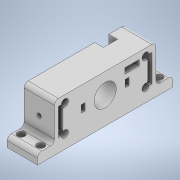
# Autodesk Inventor part: Y_motor_mount
Saved by Autodesk Inventor 2020 (Build 240168000, 168)
## iProperties
Created: 2022-04-26
Part Number: Y_motor_mount
Material: Ogólny
Document SubType Name: Modeling
Designer: mikoma
Density: 1 g/cm^3
Appearance: Domyślna
Mass: 413.903 g
Surface Area: 679.548 cm^2
Volume: 413.903 cm^3
Author: mikoma
Autodesk Inventor part; units mm, degrees
ref_plane "YZ Plane" through (0, 0, 0) normal (1, 0, 0) x (0, 1, 0)
ref_plane "XZ Plane" through (0, 0, 0) normal (0, 1, 0) x (-1, 0, 0)
ref_plane "XY Plane" through (0, 0, 0) normal (0, 0, 1) x (1, 0, 0)
sketch "Szkic1" plane through (0, 0, 0) normal (1, 0, 0) x (0, 1, 0)
  circle A0 centre (0, 0) radius 16.5
  arc A1 (16.0869, 63.5) -> (15.2371, 62.2084) centre (20, 60) ccw construction
  arc A2 (-20.25, 65.244) -> (-15.2371, 62.2084) centre (-20, 60) ccw
  line L0 (20.25, 69.5) -> (-20.25, 69.5)
  line L1 (-20.25, 69.5) -> (-20.25, 65.244)
  line L2 (-20.25, 63.5) -> (-16.0869, 63.5) construction
  line L3 (20.25, 63.5) -> (20.25, 65.244) construction
  line L4 (16.0869, 63.5) -> (20.25, 63.5) construction
  line L5 (20.25, 65.244) -> (20.25, 69.5)
  line L6 (-20.25, 65.244) -> (-20.25, 63.5) construction
  line L7 (-16.0869, 63.5) -> (-13, 63.5) construction
  arc A3 (20.25, 65.244) -> (16.0869, 63.5) centre (20, 60) ccw construction
  arc A4 (-16.0869, 63.5) -> (-20.25, 65.244) centre (-20, 60) ccw construction
  line L8 (-15.2371, 62.2084) -> (-13, 63.5)
  line L9 (13, 63.5) -> (15.2371, 62.2084)
  arc A5 (15.2371, 62.2084) -> (20.25, 65.244) centre (20, 60) ccw
  line L10 (13, 63.5) -> (16.0869, 63.5) construction
  arc A6 (-15.2371, 62.2084) -> (-16.0869, 63.5) centre (-20, 60) ccw construction
  line L11 (-13, 63.5) -> (13, 63.5)
  line L12 (16.5, 0) -> (-16.5, 0) construction
  arc A7 (15.2371, -62.2084) -> (16.0869, -63.5) centre (20, -60) ccw construction
  arc A8 (-15.2371, -62.2084) -> (-20.25, -65.244) centre (-20, -60) ccw
  line L13 (20.25, -69.5) -> (-20.25, -69.5)
  line L14 (-20.25, -69.5) -> (-20.25, -65.244)
  line L15 (-20.25, -63.5) -> (-16.0869, -63.5) construction
  line L16 (20.25, -63.5) -> (20.25, -65.244) construction
  line L17 (16.0869, -63.5) -> (20.25, -63.5) construction
  line L18 (20.25, -65.244) -> (20.25, -69.5)
  line L19 (-20.25, -65.244) -> (-20.25, -63.5) construction
  line L20 (-16.0869, -63.5) -> (-13, -63.5) construction
  arc A9 (16.0869, -63.5) -> (20.25, -65.244) centre (20, -60) ccw construction
  arc A10 (-20.25, -65.244) -> (-16.0869, -63.5) centre (-20, -60) ccw construction
  line L21 (-15.2371, -62.2084) -> (-13, -63.5)
  line L22 (13, -63.5) -> (15.2371, -62.2084)
  arc A11 (20.25, -65.244) -> (15.2371, -62.2084) centre (20, -60) ccw
  line L23 (13, -63.5) -> (16.0869, -63.5) construction
  arc A12 (-16.0869, -63.5) -> (-15.2371, -62.2084) centre (-20, -60) ccw construction
  line L24 (-13, -63.5) -> (13, -63.5)
  line L25 (24.5, 75.5) -> (-19, 75.5)
  line L26 (-40, 75.5) -> (-40, -75.5)
  line L27 (-19, -75.5) -> (24.5, -75.5)
  line L28 (30.5, -69.5) -> (30.5, -31.5)
  arc A13 (30.5, 69.5) -> (24.5, 75.5) centre (24.5, 69.5) ccw
  arc A14 (24.5, -75.5) -> (30.5, -69.5) centre (24.5, -69.5) ccw
  line L29 (-40, 75.5) -> (-25, 75.5) construction
  line L30 (-25, 81.5) -> (-25, 94.5)
  line L31 (-31, 100.5) -> (-40, 100.5)
  line L32 (-40, 100.5) -> (-40, 75.5)
  arc A15 (-25, 94.5) -> (-31, 100.5) centre (-31, 94.5) ccw
  arc A16 (-25, 81.5) -> (-19, 75.5) centre (-19, 81.5) ccw
  line L33 (-40, -75.5) -> (-25, -75.5) construction
  line L34 (-25, -81.5) -> (-25, -94.5)
  line L35 (-31, -100.5) -> (-40, -100.5)
  line L36 (-40, -100.5) -> (-40, -75.5)
  arc A17 (-31, -100.5) -> (-25, -94.5) centre (-31, -94.5) ccw
  arc A18 (-19, -75.5) -> (-25, -81.5) centre (-19, -81.5) ccw
  line L37 (30.5, 25.5) -> (30.5, -25.5) construction
  line L38 (30.5, 31.5) -> (30.5, 69.5)
  line L39 (30.5, -31.5) -> (30.5, 31.5)
  circle A19 centre (0, 0) radius 18.5
  point P0 (-25, 100.5)
  point P1 (-25, -100.5)
  dimension "d0" = 33
  dimension "d1" = 10.5
  dimension "d3" = 20
  dimension "d4" = 60
  dimension "d6" = 6
  dimension "d8" = 3.5
  dimension "d9" = 150
  dimension "d10" = 150
  dimension "d11" = 26
  dimension "d12" = 13
  dimension "d13" = 6
  dimension "d14" = 6
  dimension "d15" = 10.5
  dimension "d16" = 20
  dimension "d17" = 6
  dimension "d18" = 15
  dimension "d19" = 25
  dimension "d20" = 6
  dimension "d21" = 15
  dimension "d22" = 25
  dimension "d23" = 6
  dimension "d50" = 37
  dimension "d55" = 40
  dimension "d56" = 0.25
  dimension "d57" = 0.25
  constraints: 80 end point, 38 point on circle, 20 centre point, 14 symmetric about line, 13 parallel, 12 tangent, 11 point on line, 5 horizontal, 5 perpendicular, 4 equal radius, 2 coincident, 2 horizontal alignment, 1 collinear, 1 vertical, 6 other
  measures "d0" diameter of A0
  measures "d1" diameter of A1
  measures "d3" horizontal distance of point (0, 0) A1.centre
  measures "d4" vertical distance of A1.centre point (0, 0)
  measures "d6" distance of L3.start L0.start
  measures "d8" distance from line of L2 A1.centre
  measures "d9" angle of L8 L7
  measures "d10" angle of L7 L9
  measures "d11" distance of L7.end L9.start
  measures "d12" horizontal distance of L9.start point (0, 0)
  measures "d13" distance between parallel lines of L0 L25
  measures "d14" distance between parallel lines of L13 L27
  measures "d15" distance from line of A1.centre L28
  measures "d16" distance from line of A2.centre L26
  measures "d17" radius of A13
  measures "d18" distance of point (-25, 100.5) L31.end
  measures "d19" distance of L29.end point (-25, 100.5)
  measures "d20" radius of A15
  measures "d21" distance of point (-25, -100.5) L35.end
  measures "d22" distance of L33.end point (-25, -100.5)
  measures "d23" radius of A17
  measures "d50" diameter of A19
  measures "d55" distance of A2.centre A1.centre
  measures "d56" horizontal distance of L3.end A1.centre
  measures "d57" horizontal distance of L1.end A2.centre
extrude "Wyciągnięcie proste1" add sketch "Szkic1" along normal blind 45 contours A0 | L1 L0 L5 A5 L9 L11 L8 A2 | L21 L24 L22 A11 L18 L13 L14 A8 | A13 L38 L39 L28 A14 L27 A18 L34 A17 L35 L36 L26 L32 L31 A15 L30 A16 L25 | A19
extrude "Wyciągnięcie proste4" cut sketch "Szkic1" along normal through all contours A0 | L1 L0 L5 A5 L9 L11 L8 A2 | L21 L24 L22 A11 L18 L13 L14 A8
extrude "Wyciągnięcie proste7" cut sketch "Szkic1" along normal blind 7 contours A19
sketch "Szkic2" plane through (0, -25, 94.5) normal (0, 1, 0) x (1, 0, 0)
  circle A0 centre (37, 6.5) radius 5.5
  circle A1 centre (8, 6.5) radius 5.5
  circle A2 centre (37, 6.5) radius 3.25
  circle A3 centre (8, 6.5) radius 3.25
  line L0 (45, 13) -> (45, 0) projected
  line L1 (0, -6) -> (45, -6) projected
  line L2 (0, 13) -> (0, 0) projected
  point P0 (0, 94.5)
  dimension "d41" = 6.5
  dimension "d42" = 11
  dimension "d43" = 8
  dimension "d44" = 12.5
  dimension "d45" = 8
  constraints: 4 centre point, 2 coincident, 2 equal radius, 1 horizontal alignment
  measures "d41" diameter of A2
  measures "d42" diameter of A0
  measures "d43" distance from line of A0.centre L0
  measures "d44" distance from line of L1 A0.centre
  measures "d45" distance from line of L2 A1.centre
extrude "Wyciągnięcie proste5" cut sketch "Szkic2" against normal through all contours A2 | A3
extrude "Wyciągnięcie proste6" cut sketch "Szkic2" against normal blind 5
sketch "Szkic3" plane through (0, -19, 75.5) normal (0, 0, 1) x (1, 0, 0)
  line L0 (45, 32) -> (45, 6) projected
  line L1 (0, 32) -> (45, 32) projected
  line L2 (0, 6) -> (0, 32) projected
  line L3 (0, 6) -> (45, 6) projected
  line L4 (0, 6) -> (45, 6) projected
  line L5 (0, 32) -> (45, 6) construction
  line L6 (45, 32) -> (0, 6) construction
  circle A0 centre (22.5, 19) radius 3.25
  circle A1 centre (22.5, 19) radius 5.5
  point P0 (0, 19)
  dimension "d58" = 6.5
  dimension "d59" = 11
  constraints: 4 end point, 2 centre point, 2 midpoint, 1 coincident
  measures "d58" diameter of A0
  measures "d59" diameter of A1
extrude "Wyciągnięcie proste9" cut sketch "Szkic3" against normal blind 60 contours A0
sketch "Szkic4" plane through (45, 0, 0) normal (1, 0, 0) x (0, 0, -1)
  line L0 (-35.5, 5.25) -> (-30, 5.25)
  line L1 (-30, 5.25) -> (-30, -5.25)
  line L2 (-30, -5.25) -> (-35.5, -5.25)
  line L3 (-35.5, -5.25) -> (-35.5, 5.25)
  line L4 (-75.5, 24.5) -> (-75.5, -19) projected
  point P0 (0, 0)
  dimension "d62" = 10.5
  dimension "d63" = 5.25
  dimension "d64" = 40
  dimension "d65" = 5.5
  constraints: 8 end point, 2 parallel, 1 horizontal, 1 perpendicular
  measures "d62" distance of L0.end L1.end
  measures "d63" distance from line of point (0, 0) L0
  measures "d64" distance between parallel lines of L4 L3
  measures "d65" distance between parallel lines of L3 L1
extrude "Wyciągnięcie proste10" cut sketch "Szkic4" against normal blind 28.75
mirror "Odbij3" about plane through (0, 0, 0) normal (0, 0, 1) of "Wyciągnięcie proste10", "Wyciągnięcie proste9", "Wyciągnięcie proste6", "Wyciągnięcie proste5"
sketch "Szkic5" plane through (0, 30.5, 69.5) normal (0, 1, 0) x (1, 0, 0)
  line L0 (0, 51) -> (0, 88) projected
  line L1 (0, 124.25) -> (0, 134.744) projected
  line L2 (0, -31) -> (0, 170) projected
  line L3 (0, 120) -> (13, 120)
  line L4 (13, 120) -> (13, 99)
  line L5 (13, 99) -> (0, 99)
  line L6 (0, 99) -> (0, 120)
  point P0 (0, 69.5)
  point P1 (0, 131.7084)
  point P2 (0, 99)
  dimension "d68" = 21
  dimension "d69" = 13
  dimension "d70" = 11
  constraints: 8 end point, 2 parallel, 1 horizontal, 1 perpendicular, 2 other
  measures "d68" distance of L3.end L4.end
  measures "d69" distance of L4.end L5.end
  measures "d70" distance of L5.end L0.end
extrude "Wyciągnięcie proste11" cut sketch "Szkic5" against normal blind 18
sketch "Szkic6" plane through (13, 30.5, -50.5) normal (-1, 0, 0) x (0, 0, 1)
  line L0 (21, -18) -> (0, -18) projected
  line L1 (21, 0) -> (21, -18) projected
  line L2 (0, -18) -> (21, -18)
  line L3 (21, -18) -> (21, -10)
  line L4 (21, -10) -> (0, -10)
  line L5 (0, -10) -> (0, -18)
  point P0 (50.5, -30.5)
  dimension "d74" = 8
  constraints: 8 end point, 2 parallel, 1 horizontal, 1 perpendicular, 1 point on line
  measures "d74" distance of L4.end L0.end
extrude "Wyciągnięcie proste12" cut sketch "Szkic6" against normal through all
sketch "Szkic7" plane through (0, 12.5, 69.5) normal (0, 1, 0) x (1, 0, 0)
  circle A0 centre (8.5, 114.5) radius 1.75
  circle A1 centre (8.5, 104.5) radius 1.75
  line L0 (0, 120) -> (13, 120) projected
  line L1 (0, 99) -> (0, 120) projected
  point P0 (0, 69.5)
  dimension "d77" = 5.5
  dimension "d78" = 10
  dimension "d79" = 3.5
  dimension "d80" = 8.5
  constraints: 2 centre point, 1 equal radius, 1 vertical alignment
  measures "d77" distance from line of L0 A0.centre
  measures "d78" distance of A0.centre A1.centre
  measures "d79" diameter of A1
  measures "d80" distance from line of L1 A1.centre
extrude "Wyciągnięcie proste13" cut sketch "Szkic7" against normal through all
sketch "Szkic10" plane through (0, 0, 0) normal (-1, 0, 0) x (0, 0, 1)
  line L0 (-46.75, 12.5) -> (-43.25, 12.5) projected
  line L1 (-36.75, 12.5) -> (-33.25, 12.5) projected
  line L2 (-48, 6) -> (-42, 6)
  line L3 (-42, 6) -> (-42, 3.4)
  line L4 (-42, 3.4) -> (-48, 3.4)
  line L5 (-48, 3.4) -> (-48, 6)
  line L6 (-38, 6) -> (-32, 6)
  line L7 (-32, 6) -> (-32, 3.4)
  line L8 (-32, 3.4) -> (-38, 3.4)
  line L9 (-38, 3.4) -> (-38, 6)
  line L10 (-29.5, 12.5) -> (-50.5, 12.5) projected
  line L11 (-50.5, 12.5) -> (-50.5, 30.5) projected
  point P0 (0, 0)
  dimension "d83" = 6.5
  dimension "d84" = 2.6
  dimension "d85" = 6
  dimension "d86" = 6
  dimension "d87" = 2.5
  dimension "d89" = 10
  constraints: 16 end point, 4 parallel, 2 horizontal, 2 perpendicular, 2 point on line
  measures "d83" distance between parallel lines of L10 L2
  measures "d84" distance of L4.end L2.start
  measures "d85" distance of L3.end L4.end
  measures "d86" distance of L6.start L6.end
  measures "d87" distance between parallel lines of L11 L5
  measures "d89" distance between parallel lines of L9 L5
extrude "Wyciągnięcie proste14" cut sketch "Szkic10" against normal blind 11
equation "\"d3\" = 0.5 * d2"
equation "\"d12\" = 0.5 * d11"
equation "\"d14\" = d13"
equation "\"d2\" = 40"
